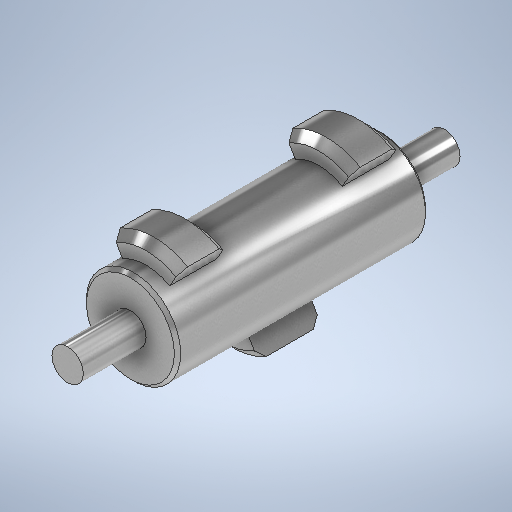
# Autodesk Inventor part: Part3
Saved by Autodesk Inventor 2025 (Build 290162000, 162)
## iProperties
Created: 2026-06-07
Part Number: Part3
Material: Generic
Document SubType Name: Modeling
Designer: user
Density: 1 g/cm^3
Appearance: Honed
Author: user
Autodesk Inventor part; units mm, degrees
ref_plane "YZ Plane" through (0, 0, 0) normal (1, 0, 0) x (0, 1, 0)
sketch "Sketch1" plane through (0, 0, 0) normal (0, 0, 1) x (1, 0, 0)
  circle A0 centre (0, 0) radius 30
  dimension "d0" = 60
  constraints: 1 centre point, 1 coincident
  measures "d0" diameter of A0
extrude "Extrusion1" add sketch "Sketch1" along normal blind 160
ref_plane "Work Plane1" through (0, 0, 150) normal (0, 0, 1) x (1, 0, 0)
sketch "Sketch4" plane through (0, 0, 150) normal (0, 0, 1) x (1, 0, 0)
  circle A0 centre (0, 0) radius 30 projected
  line L0 (0, 0) -> (21.5, 37.2391)
  line L1 (0, 0) -> (43, 0) construction
  line L2 (0, 0) -> (-25, 43.3013)
  arc A1 (21.5, 37.2391) -> (-21.5, 37.2391) centre (0, 0) ccw
  point P0 (-21.5, 37.2391)
  point P1 (-15, 25.9808)
  point P2 (15, 25.9808)
  dimension "d6" = 43
  dimension "d7" = 60
  constraints: 6 end point, 2 point on circle, 1 centre point, 1 coincident, 1 equal length, 1 horizontal
  measures "d6" distance of L0.start L0.end
  measures "d7" angle of L1 L0
extrude "Extrusion2" add sketch "Sketch4" against normal blind 30 contours A0 L2 A1 L0
ref_plane "Work Plane2" through (0, 0, 80) normal (0, 0, 1) x (1, 0, 0)
mirror "Mirror1" about plane through (0, 0, 80) normal (0, 0, 1) of "Extrusion2"
sketch "Sketch5" plane through (0, 0, 80) normal (0, 0, 1) x (1, 0, 0)
  line L0 (0, 0) -> (21.5, -37.2391)
  line L1 (0, 0) -> (43, 0) construction
  circle A0 centre (0, 0) radius 30 projected
  line L2 (0, 0) -> (-21.5, -37.2391)
  arc A1 (-21.5, -37.2391) -> (21.5, -37.2391) centre (0, 0) ccw
  point P0 (15, -25.9808)
  point P1 (-15, -25.9808)
  dimension "d10" = 43
  dimension "d11" = 60
  constraints: 6 end point, 2 point on circle, 1 centre point, 1 coincident, 1 equal length, 1 horizontal
  measures "d10" distance of L0.start L0.end
  measures "d11" angle of L0 L1
extrude "Extrusion3" add sketch "Sketch5" along normal mid plane 40 contours L0 A1 L2 A0
chamfer "Chamfer1" distance 5 angle 45 6 edges at (0, 43, 150) (0, 43, 120) (0, 43, 40) (0, 43, 10) (0, -43, 100) (0, -43, 60)
chamfer "Chamfer2" distance 2 angle 45 2 edges at (-30, 0, 0) (-30, 0, 160)
sketch "Sketch6" plane through (0, 0, 160) normal (0, 0, 1) x (1, 0, 0)
  circle A0 centre (0, 0) radius 10
  dimension "d20" = 20
  constraints: 1 centre point, 1 coincident
  measures "d20" diameter of A0
extrude "Extrusion4" add sketch "Sketch6" along normal blind 40 and the other way blind 200
body "Solid1"
